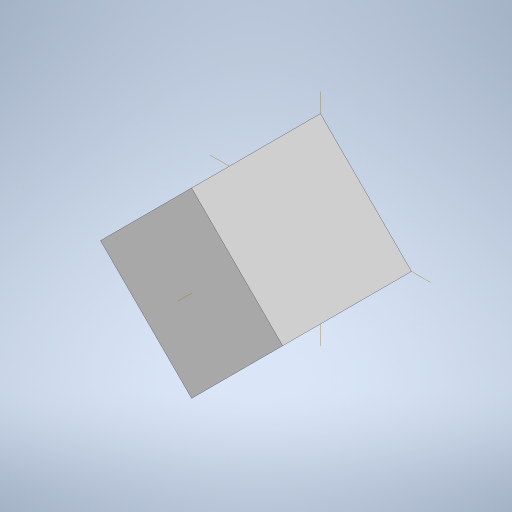
# Autodesk Inventor part: Cube
Saved by Autodesk Inventor 2023.2 (Build 272271030, 271C)
## iProperties
Created: 2023-02-16
Part Number: Cube
Material: Generisch
Document SubType Name: Modeling
Designer: mehan
Density: 1 g/cm^3
Appearance: Vorgabe
Author: mehan
Autodesk Inventor part; units mm, degrees
ref_plane "YZ Plane" through (0, 0, 0) normal (1, 0, 0) x (0, 1, 0)
ref_plane "XZ Plane" through (0, 0, 0) normal (0, 1, 0) x (-1, 0, 0)
ref_plane "XY Plane" through (0, 0, 0) normal (0, 0, 1) x (1, 0, 0)
sketch "Skizze1" plane through (0, 0, 0) normal (0, 0, 1) x (1, 0, 0)
  line L0 (0, -35.3553) -> (35.3553, 0)
  line L1 (35.3553, 0) -> (0, 35.3553)
  line L2 (0, 35.3553) -> (-35.3553, 0)
  line L3 (-35.3553, 0) -> (0, -35.3553)
  line L4 (0, -35.3553) -> (0, 35.3553) construction
  line L5 (35.3553, 0) -> (-35.3553, 0) construction
  line L6 (0, -35.3553) -> (50, -35.3553) construction
  point P0 (0, 0)
  dimension "d0" = 50
  dimension "d1" = 45
  dimension "d2" = 50
  constraints: 14 end point, 2 midpoint, 2 parallel, 1 equal length, 1 horizontal, 1 perpendicular
  measures "d0" distance of L0.start L0.end
  measures "d1" angle of L6 L0
  measures "d2" distance of L1.end L0.end
extrude "Extrusion1" add sketch "Skizze1" along normal blind 50
